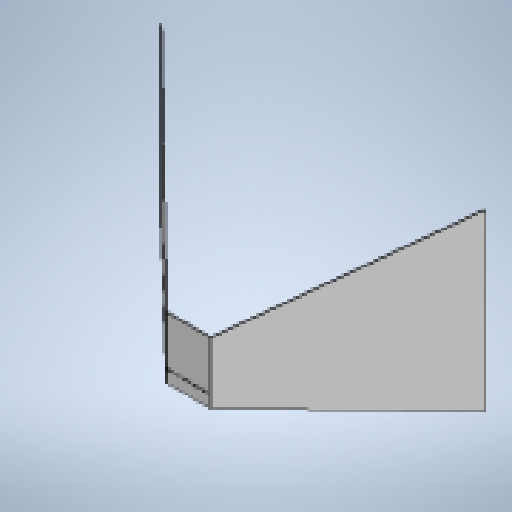
# Autodesk Inventor part: MSC 505 sheet belly-neck
Saved by Autodesk Inventor 2025 (Build 290162010, 162A)
## iProperties
Created: 2024-04-28
Part Number: MSC 505 sheet belly-neck
Material: Stainless Steel
Document SubType Name: Sheet Metal
Designer: admin
Stock Number: МОО 502 лист брюхо-горло
Mass: 38113.6 g
Surface Area: 31958.5 cm^2
Volume: 4764.2 cm^3
Density: 8 g/cm^3
Flat Pattern Width: 79.7119 cm
Flat Pattern Length: 88.7 cm
Flat Pattern Area: 7070.45 cm^2
Sheet Metal Rule: Default_mm
Sheet Metal Width: 797,119 mm
Sheet Metal Length: 887,000 mm
Sheet Metal Area: 707044,555 mm^2
Appearance: Default
Author: admin
Autodesk Inventor part; units mm, degrees
ref_plane "YZ Plane" through (0, 0, 0) normal (1, 0, 0) x (0, 1, 0)
ref_plane "XZ Plane" through (0, 0, 0) normal (0, 1, 0) x (-1, 0, 0)
ref_plane "XY Plane" through (0, 0, 0) normal (0, 0, 1) x (1, 0, 0)
sketch "Sketch1" plane through (0, 0, 0) normal (0, 0, 1) x (1, 0, 0)
  arc A0 (100, 0) -> (104.168, 1.684) centre (100, 6) ccw
  line L0 (104.168, 1.684) -> (742.2224, 617.8459)
  line L1 (0, 0) -> (100, 0)
  dimension "d73" = 6
  dimension "d74" = 742.2224
  dimension "d75" = 136
  dimension "d76" = 100
  dimension "d82" = 887
  measures "d73" radius of A0
  measures "d74" horizontal distance of L1.start L0.end
  measures "d75" angle of L1 L0
  measures "d76" distance of L1.start L1.end
  measures "d82" distance of L0.start L0.end
contour flange "Contour Flange1" sketch "Sketch1" thickness 3 bend radius 3 width 800 along (0, 0, 1) mid plane no both sides no wall seen from (50, 0, 0) lies toward (0, 1, 0) curves L1 A0 L0
bend "Bend1"
corner "Corner1"
mirror "Mirror1" about plane through (0, 0, 0) normal (1, 0, 0)
sketch "Sketch7" plane through (-104.168, 1.684, 0) normal (0, 0, -1) x (-0.7193398, 0.6946584, 0)
  line L0 (0, 0) -> (0, 3) projected
  line L1 (0, 0) -> (-233.6012, 0)
  line L2 (-233.6012, 0) -> (-233.6012, 1093.4776)
  line L3 (-233.6012, 1093.4776) -> (0, 1093.4776)
  line L4 (0, 1093.4776) -> (0, 0)
  point P0 (-76.1019, 71.1498)
  point P1 (0, 3)
  constraints: 8 end point, 2 parallel, 1 horizontal, 1 perpendicular
sketch "Sketch2" plane through (0, 0, 0) normal (1, 0, 0) x (0, 1, 0)
  line L0 (620.004, 0) -> (620.004, 800) projected
  line L1 (0, 800) -> (0, 0) projected
  line L2 (620.004, 800) -> (0, 800)
  line L3 (620.004, 800) -> (0, 279.7549)
  dimension "d81" = 40
  constraints: 4 end point, 1 perpendicular, 1 point on line
  measures "d81" angle of L2 L3
extrude "Extrusion1" cut sketch "Sketch2" along normal through all both and the other way through all
fillet "Fillet1" radius 4 2 edges at (741.1804, 618.9249, 799.0946) (-741.1804, 618.9249, 799.0946)
extrude "Extrusion3" cut sketch "Sketch7" along normal through all both and the other way through all
sketch "Sketch8" plane through (-740.1384, 620.004, 792.4468) normal (0.6946584, 0.7193398, 0) x (0.7193398, -0.6946584, 0)
  line L0 (27.1118, 77.5366) -> (27.1118, 257.5454) construction
  line L1 (27.1118, 257.5454) -> (33.3302, 257.5454) construction
  line L2 (33.3302, 257.5454) -> (33.3302, 77.5366) construction
  line L3 (33.3302, 77.5366) -> (27.1118, 77.5366) construction
  point P0 (963.1019, 792.4468)
  constraints: 2 other
mark "Mark2"
equation "\"d7\" = Thickness"
equation "\"d8\" = BendReliefWidth"
equation "\"d9\" = BendReliefDepth"
equation "\"d10\" = MinimumRemnant"
equation "\"d11\" = TransitionRadius"
equation "\"d13\" = BendRadius"
equation "\"d15\" = CornerReliefSize"
equation "\"d16\" = GapSize"
equation "\"d17\" = JacobiRadiusSize"
equation "\"BendRadius\" = Thickness"
equation "\"BendReliefWidth\" = Thickness"
equation "\"BendReliefDepth\" = 0.5 * Thickness"
equation "\"CornerReliefSize\" = 4 * Thickness"
equation "\"MinimumRemnant\" = 2 * Thickness"
equation "\"TransitionRadius\" = BendRadius"
equation "\"JacobiRadiusSize\" = BendRadius"
equation "\"GapSize\" = Thickness"
equation "\"d38\" = d40 + d44"
equation "\"d39\" = d40"
equation "\"d44\" = d40"
equation "\"Thickness\" = 3"
equation "\"d40\" = 3"
body "Solid1"
